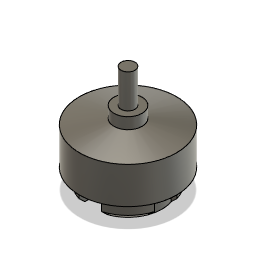
Main_Bar v2 (Autodesk Fusion 360 archive; units mm, degrees)
design "AX2810Q750kv v1"
Autodesk Fusion 360 part; units mm, degrees
sketch "Skizze3" plane through (0, 0, 0) normal (0, 0, 1) x (1, 0, 0)
  line L0 (5, 26) -> (5, 22)
  line L1 (5, 22) -> (17.25, 20)
  line L2 (17.25, 20) -> (17.25, 7)
  line L3 (17.25, 7) -> (15, 7)
  line L4 (15, 7) -> (15, 6)
  line L5 (15, 6) -> (14, 6)
  line L6 (14, 6) -> (14, 2)
  line L7 (14, 2) -> (12, 0)
  line L8 (12, 0) -> (0, 0)
  line L9 (0, 0) -> (0, 26)
  line L10 (0, 26) -> (5, 26)
  line L11 (0, 26) -> (2.5, 26)
  line L12 (2.5, 26) -> (2.5, 38)
  line L13 (2.5, 38) -> (0, 38)
  line L14 (0, 38) -> (0, 26)
  line L15 (17.25, 7) -> (0, 7)
  line L16 (0, 7) -> (0, 18.5)
  line L17 (0, 18.5) -> (17.25, 18.5)
  line L18 (17.25, 18.5) -> (17.25, 7)
  dimension "d4" = 26
  dimension "d5" = 4
  dimension "d6" = 17.25
  dimension "d7" = 12
  dimension "d8" = 14
  dimension "d9" = 1
  dimension "d12" = 45
  dimension "d13" = 5
  dimension "d14" = 2.5
  dimension "d15" = 12
  dimension "d16" = 2
  dimension "d17" = 1
  dimension "d18" = 6
  dimension "d19" = 1.5
  constraint vertical L0
  constraint parallel L0 L2
  constraint perpendicular L2 L3
  constraint perpendicular L3 L4
  constraint perpendicular L4 L5
  constraint perpendicular L5 L6
  constraint perpendicular L4 L8
  constraint perpendicular L8 L9
  constraint horizontal L11
  constraint vertical L12
  constraint horizontal L13
  constraint vertical L14
  constraint coincident L8.end L9.start
  constraint horizontal L15
  constraint vertical L16
  constraint horizontal L17
  constraint vertical L18
  constraint coincident L9 L16.end
  measures "d4" distance of L8 L10
  measures "d5" distance of L0.start L0.end
  measures "d6" distance of L2 L9
  measures "d7" distance of L7.end L8.end
  measures "d8" distance of L6 L9
  measures "d9" distance of L4 L6
  measures "d12" angle of L7 L8
  measures "d13" distance of L0 L9
  measures "d14" distance of L12 L14
  measures "d15" distance of L10 L13
  measures "d16" vertical distance of L0.end L1.end
  measures "d17" distance of L3.end L4.end
  measures "d18" distance of L5 L8
  measures "d19" distance of L1.end L17
revolve "Drehen1" add sketch "Skizze3" angle 360 about axis through (0, 0, 0) along (0, 1, 0)
sketch "Skizze4" plane through (0, 0, 0) normal (0, -1, 0) x (1, 0, 0)
  circle A0 centre (0, 0) radius 12
  circle A1 centre (0, 0) radius 12 construction
  circle A2 centre (0, 0) radius 14 construction
  circle A3 centre (0, 0) radius 14
  line L0 (-4, 14) -> (4, 14) construction
  line L1 (4, 14) -> (4, 8)
  line L2 (4, 8) -> (-4, 8)
  line L3 (-4, 8) -> (-4, 14)
  circle A4 centre (-5.6569, 5.6569) radius 1.5
  circle A5 centre (5.6569, -5.6569) radius 1.5
  circle A6 centre (-6.7175, -6.7175) radius 1.5
  circle A7 centre (6.7175, 6.7175) radius 1.5
  line L4 (-5.6569, 5.6569) -> (5.6569, -5.6569) construction
  line L5 (6.7175, 6.7175) -> (-6.7175, -6.7175) construction
  line L6 (-8, -4) -> (-14, -4)
  line L7 (-8, 4) -> (-8, -4)
  line L8 (-14, 4) -> (-8, 4)
  line L9 (4, -8) -> (4, -14)
  line L10 (-4, -8) -> (4, -8)
  line L11 (-4, -14) -> (-4, -8)
  line L12 (8, 4) -> (14, 4)
  line L13 (8, -4) -> (8, 4)
  line L14 (14, -4) -> (8, -4)
  dimension "d21" = 28
  dimension "d22" = 8
  dimension "d23" = 4
  dimension "d24" = 6
  dimension "d28" = 3
  dimension "d31" = 16
  dimension "d32" = 19
  dimension "d33" = 9.5
  dimension "d35" = 8
  dimension "d36" = 45
  dimension "d38" = 360
  constraint coincident A0.centre A1.centre
  constraint horizontal L0
  constraint vertical L1
  constraint horizontal L2
  constraint vertical L3
  constraint tangent A3 L0
  constraint equal A4 A7
  constraint equal A4 A5
  constraint equal A4 A6
  constraint coincident A4.centre L4.start
  constraint coincident A5.centre L4.end
  constraint coincident A7.centre L5.start
  constraint coincident A6.centre L5.end
  constraint perpendicular L4 L5
  constraint coincident A0.centre L5
  constraint coincident A0.centre L4
  measures "d21" diameter of A3
  measures "d22" distance of L1.end L2.end
  measures "d23" distance of A0.centre L1
  measures "d24" distance of L0.end L1.end
  measures "d28" diameter of A4
  measures "d31" distance of A4.centre A5.centre
  measures "d32" distance of A7.centre A6.centre
  measures "d33" distance of A0.centre A7.centre
  measures "d35" distance of A0.centre A5.centre
  measures "d36" angle of L2 L5
extrude "Extrusion2" cut sketch "Skizze4" against normal blind 6 contours A0 A3 L12 L14 | A0 L1 L2 L3 | A0 A3 L1 L3 | A0 A3 L9 L11 | A0 L9 L10 L11 | A0 L6 L7 L8 | A0 A3 L6 L8 | A4 | A5 | A6 | A7
equation "d6 = ( 34.5 / 2 ) * 1 mm"
equation "d23 = d22 / 2"
equation "d33 = d32 / 2"
equation "d35 = d31 / 2"
